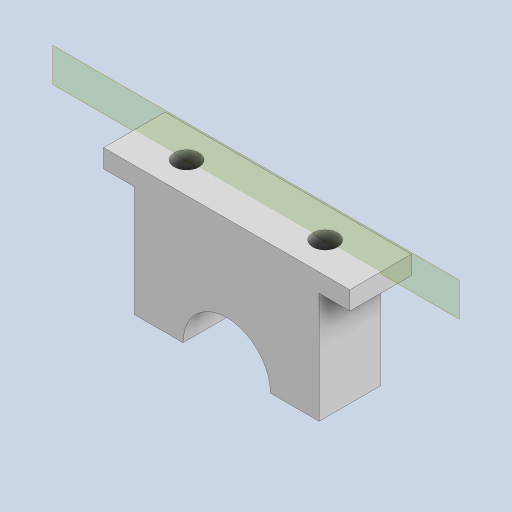
# Autodesk Inventor part: цили
Saved by Autodesk Inventor 2024.2 (Build 282272000, 272)
## iProperties
Created: 2025-11-23
Part Number: цили
Material: Типовые
Document SubType Name: Modeling
Designer: katya_notebook
Density: 1 g/cm^3
Appearance: По умолчанию
Author: katya_notebook
Autodesk Inventor part; units mm, degrees
ref_plane "YZ Plane" through (0, 0, 0) normal (1, 0, 0) x (0, 1, 0)
ref_plane "XZ Plane" through (0, 0, 0) normal (0, 1, 0) x (-1, 0, 0)
ref_plane "XY Plane" through (0, 0, 0) normal (0, 0, 1) x (1, 0, 0)
ref_plane "РабПлоскость2" through (-434.0611, 188.1702, -199.3103) normal (0, 0, -1) x (-1, 0, 0)
sketch "Эскиз2" plane through (-434.0611, 188.1702, -199.3103) normal (0, 0, -1) x (-1, 0, 0)
  circle A0 centre (-30.2445, -26) radius 2.5 projected
  circle A1 centre (-30.2445, -26) radius 2.5
  circle A2 centre (-30.2445, -26) radius 7.1
  line L0 (-60, -5) -> (0, -5) projected
  line L1 (-30.2445, -26) -> (-30.2445, -50.8115)
  line L2 (-30.2445, -50.8115) -> (-30.2445, 7.1034)
  line L3 (-30.2445, -5) -> (-50.2445, -5)
  line L4 (-50.2445, -5) -> (-50.2445, -8)
  line L5 (-50.2445, -8) -> (-45.2445, -8)
  circle A3 centre (-30.2445, -26) radius 15
  line L6 (-45.2445, -26) -> (-45.2445, -8)
  line L7 (-45.2445, -26) -> (-30.2445, -26)
  line L8 (-30.2445, -5) -> (-10.2445, -5)
  line L9 (-10.2445, -5) -> (-10.2445, -8)
  line L10 (-10.2445, -8) -> (-15.2445, -8)
  line L11 (-15.2445, -26) -> (-15.2445, -8)
  line L12 (-15.2445, -26) -> (-30.2445, -26)
  point P0 (-434.0611, -188.1702)
  point P1 (-37.3445, -26)
  point P2 (-23.1445, -26)
  point P3 (-10.2445, -5)
  dimension "d5" = 30
  dimension "d1" = 14.2
  dimension "d2" = 20
  dimension "d3" = 3
  constraints: 24 end point, 4 point on line, 4 symmetric about line, 3 coincident, 3 vertical, 2 centre point, 2 horizontal, 1 concentric, 1 horizontal alignment, 2 other
  measures "d1" diameter of A2
  measures "d2" distance of L3.start L3.end
  measures "d3" distance of L3.end L4.end
extrude "Выдавливание1" add sketch "Эскиз2" along normal mid plane 10 contours A2 L2 A3 L12 | A2 L7 A3 L2 | A3 L2 L0 L9 L10 L11 | A3 L6 L5 L4 L0 L2
sketch "Эскиз3" plane through (-396.7166, 162.1702, -204.3103) normal (0, -1, 0) x (1, 0, 0)
  spline S0 degree 3 poles (5.9, 5) (5.9, 4.8797) (5.8891, 4.7613) (5.8484, 4.5339) (5.8186, 4.4249) (5.7083, 4.1184) (5.606, 3.9413) (5.2388, 3.4516) (4.8957, 3.2183) (4.1196, 2.9708) (3.6855, 2.9633) (3.0889, 3.1622) (2.8946, 3.2566) (2.5333, 3.5227) (2.3666, 3.695) (2.1389, 4.0357) (2.0497, 4.2145) (1.9301, 4.5998) (1.9, 4.8065) (1.9, 5.1935) (1.9301, 5.4002) (2.0497, 5.7855) (2.1389, 5.9643) (2.3666, 6.305) (2.5333, 6.4773) (2.8946, 6.7434) (3.0889, 6.8378) (3.6855, 7.0367) (4.1196, 7.0292) (4.8957, 6.7817) (5.2388, 6.5484) (5.606, 6.0587) (5.7083, 5.8816) (5.8186, 5.5751) (5.8484, 5.4661) (5.8891, 5.2387) (5.9, 5.1203) (5.9, 5) knots 0 0 0 0 0.036086 0.036086 0.072173 0.072173 0.144346 0.144346 0.322747 0.322747 0.501149 0.501149 0.577509 0.577509 0.653869 0.653869 0.711915 0.711915 0.769961 0.769961 0.828007 0.828007 0.886052 0.886052 0.962412 0.962412 1.038772 1.038772 1.217174 1.217174 1.395575 1.395575 1.467748 1.467748 1.503835 1.503835 1.539921 1.539921 1.539921 1.539921 projected
  spline S1 degree 3 poles (-16.6168, 5) (-16.6168, 4.8248) (-16.6415, 4.6369) (-16.7405, 4.2837) (-16.8145, 4.1184) (-17.0043, 3.798) (-17.1448, 3.6306) (-17.4526, 3.3609) (-17.6194, 3.2581) (-18.1541, 3.0096) (-18.5583, 2.966) (-19.2988, 3.0829) (-19.6353, 3.2426) (-20.1233, 3.6543) (-20.3476, 3.9317) (-20.5191, 4.3736) (-20.5546, 4.4889) (-20.6036, 4.7379) (-20.6168, 4.8721) (-20.6168, 5.1279) (-20.6036, 5.2621) (-20.5546, 5.5111) (-20.5191, 5.6264) (-20.3476, 6.0683) (-20.1233, 6.3457) (-19.6353, 6.7574) (-19.2988, 6.9171) (-18.5583, 7.034) (-18.1541, 6.9904) (-17.6194, 6.7419) (-17.4526, 6.6391) (-17.1448, 6.3694) (-17.0043, 6.202) (-16.8145, 5.8816) (-16.7405, 5.7163) (-16.6415, 5.3631) (-16.6168, 5.1752) (-16.6168, 5) knots 0 0 0 0 0.052568 0.052568 0.105137 0.105137 0.174601 0.174601 0.244066 0.244066 0.414781 0.414781 0.585496 0.585496 0.721852 0.721852 0.760221 0.760221 0.798591 0.798591 0.83696 0.83696 0.875329 0.875329 1.011685 1.011685 1.1824 1.1824 1.353115 1.353115 1.42258 1.42258 1.492044 1.492044 1.544613 1.544613 1.597181 1.597181 1.597181 1.597181 projected
  point P0 (396.7166, 204.3103)
  point P1 (5.9, 5)
  point P2 (-16.6168, 5)
extrude "Выдавливание2" cut sketch "Эскиз3" against normal blind 30.25
